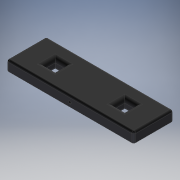
# Autodesk Inventor part: ButtonMount
Saved by Autodesk Inventor 2018 (Build 220112000, 112)
## iProperties
Created: 2018-05-19
Part Number: ButtonMount
Material: Generic
Document SubType Name: Modeling
Designer: reide
Density: 1 g/cm^3
Appearance: Default
Author: reide
Autodesk Inventor part; units mm, degrees
ref_plane "YZ Plane" through (0, 0, 0) normal (1, 0, 0) x (0, 1, 0)
ref_plane "XZ Plane" through (0, 0, 0) normal (0, 1, 0) x (-1, 0, 0)
ref_plane "XY Plane" through (0, 0, 0) normal (0, 0, 1) x (1, 0, 0)
sketch "Sketch1" plane through (0, 0, 0) normal (0, 0, 1) x (1, 0, 0)
  arc A0 (-6.8536, -19) -> (-5.8536, -20) centre (-5.8536, -19) ccw projected
  line L0 (-5.8536, -20) -> (5.8536, -20) projected
  line L1 (6.8536, -19) -> (6.8536, 19) projected
  line L2 (5.8536, 20) -> (-5.8536, 20) projected
  arc A1 (-5.8536, 20) -> (-6.8536, 19) centre (-5.8536, 19) ccw projected
  line L3 (-6.8536, 19) -> (-6.8536, -19) projected
  line L4 (-120.2387, -20) -> (-108.5315, -20) projected
  arc A2 (-108.5315, -20) -> (-107.5315, -19) centre (-108.5315, -19) ccw projected
  line L5 (-107.5315, -19) -> (-107.5315, 19) projected
  arc A3 (-107.5315, 19) -> (-108.5315, 20) centre (-108.5315, 19) ccw projected
  line L6 (-108.5315, 20) -> (-120.2387, 20) projected
  line L7 (-121.2387, 19) -> (-121.2387, -19) projected
  line L8 (-5.8536, 20) -> (-108.5315, 20)
  line L9 (-108.5315, -20) -> (-5.8536, -20)
  arc A4 (-119.2387, 20) -> (-121.2387, 18) centre (-119.2387, 18) ccw
  arc A5 (-121.2387, -18) -> (-119.2387, -20) centre (-119.2387, -18) ccw
  arc A6 (6.8536, 18) -> (4.8536, 20) centre (4.8536, 18) ccw
  arc A7 (4.8536, -20) -> (6.8536, -18) centre (4.8536, -18) ccw
  line L10 (4.8536, 20) -> (-119.2387, 20)
  line L11 (-119.2387, 20) -> (-119.2387, -20)
  line L12 (-119.2387, -20) -> (4.8536, -20)
  line L13 (4.8536, -20) -> (4.8536, 20)
  point P0 (0, 0)
  point P1 (-37.707, 3.5151)
  constraints: 12 end point, 8 point on circle, 4 centre point, 2 parallel, 2 point on line, 1 horizontal, 1 perpendicular, 17 other
extrude "Extrusion1" add sketch "Sketch1" along normal blind 10
sketch "Sketch2" plane through (0, 0, 10) normal (0, 0, 1) x (1, 0, 0)
  line L0 (6.8536, -18) -> (6.8536, 18) projected
  line L1 (-119.2387, -20) -> (4.8536, -20) projected
  line L2 (-57.1926, 0) -> (-27.1926, 0)
  line L3 (-27.1926, 0) -> (-87.1926, 0)
  line L4 (-27.1926, 0) -> (-27.1926, -5.1)
  line L5 (-27.1926, -5.1) -> (-16.9926, -5.1)
  line L6 (-16.9926, -5.1) -> (-16.9926, 5.1)
  line L7 (-16.9926, 5.1) -> (-27.1926, 5.1)
  line L8 (-27.1926, 5.1) -> (-27.1926, -5.1)
  line L9 (-57.1926, 0) -> (-57.1926, -20)
  line L10 (-57.1926, 0) -> (-87.1926, 0)
  line L11 (-87.1926, 0) -> (-27.1926, 0)
  line L12 (-87.1926, 0) -> (-87.1926, -5.1)
  line L13 (-87.1926, -5.1) -> (-97.3926, -5.1)
  line L14 (-97.3926, -5.1) -> (-97.3926, 5.1)
  line L15 (-97.3926, 5.1) -> (-87.1926, 5.1)
  line L16 (-87.1926, 5.1) -> (-87.1926, -5.1)
  point P0 (0, 0)
  point P1 (6.8536, 0)
  point P2 (6.8536, -19)
  point P3 (6.8536, 19)
  point P4 (-120.2387, -20)
  point P5 (5.8536, -20)
  dimension "d4" = 30
  dimension "d5" = 60
  dimension "d6" = 5.1
  dimension "d7" = 10.2
  dimension "d8" = 10.2
  constraints: 30 end point, 6 symmetric about line, 2 horizontal, 2 midpoint, 2 parallel, 2 point on line, 2 vertical, 1 perpendicular
  measures "d4" distance of L2.start L2.end
  measures "d5" distance of L2.end L3.end
  measures "d6" distance of L2.end L4.end
  measures "d7" distance of L4.end L5.end
  measures "d8" distance of L7.end L4.end
extrude "Extrusion2" cut sketch "Sketch2" against normal blind 100
fillet "Fillet1" radius 2 4 edges at (-57.1926, -20, 10) (6.8536, 0, 10) (-57.1926, 20, 10) (-121.2387, 0, 10)
sketch "Sketch4" plane through (-119.2387, 20, 0) normal (0, 1, 0) x (1, 0, 0)
  line L0 (124.0922, -8) -> (0, -8) projected
  line L1 (124.0922, 0) -> (124.0922, -8) projected
  line L2 (124.0922, 0) -> (0, 0) projected
  line L3 (0, 0) -> (0, -8) projected
  line L4 (60.0461, -21.2353) -> (60.0461, 6.8237)
  line L5 (63.5461, 6.8237) -> (63.5461, -21.2353)
  arc A0 (60.0461, -21.2353) -> (63.5461, -21.2353) centre (61.7961, -21.2353) ccw
  circle A1 centre (61.7961, -4) radius 1.4
  point P0 (119.2387, 0)
  dimension "d13" = 2.8
  constraints: 4 end point, 2 centre point, 2 point on circle, 2 vertical, 6 other
  measures "d13" diameter of A1
extrude "Extrusion3" cut sketch "Sketch4" against normal blind 8 contours A1
sketch "Sketch5" plane through (-119.2387, -20, 0) normal (0, -1, 0) x (1, 0, 0)
  circle A0 centre (61.7961, 26.2353) radius 1.75
  line L0 (0, 8) -> (124.0922, 8) projected
  line L1 (0, 0) -> (0, 8) projected
  line L2 (0, 0) -> (124.0922, 0) projected
  line L3 (124.0922, 0) -> (124.0922, 8) projected
  circle A1 centre (61.7961, 4) radius 1.4 projected
  circle A2 centre (61.7961, 4) radius 1.6
  point P0 (119.2387, 0)
  constraints: 2 centre point, 1 coincident, 2 other
extrude "Extrusion4" cut sketch "Sketch5" against normal blind 8 contours A1
fillet "Fillet2" radius 4 8 edges at (-92.2926, 5.1, 10) (-87.1926, 0, 10) (-92.2926, -5.1, 10) (-97.3926, 0, 10) (-22.0926, 5.1, 10) (-16.9926, 0, 10) (-27.1926, 0, 10) (-22.0926, -5.1, 10)
fillet "Fillet3" radius 2 8 edges at (-92.2926, -5.1, 0) (-97.3926, 0, 0) (-92.2926, 5.1, 0) (-87.1926, 0, 0) (-22.0926, -5.1, 0) (-16.9926, 0, 0) (-22.0926, 5.1, 0) (-27.1926, 0, 0)
body "Solid1"
